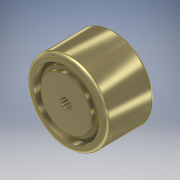
# Autodesk Inventor part: Kolo
Saved by Autodesk Inventor 2017 (Build 210142000, 142)
## iProperties
Created: 2016-11-09
Part Number: Kolo
Material: Generic
Document SubType Name: Modeling
Designer: Shichi
Density: 1 g/cm^3
Appearance: Gold - Metal
Author: Shichi
Autodesk Inventor part; units mm, degrees
ref_plane "YZ Plane" through (0, 0, 0) normal (1, 0, 0) x (0, 1, 0)
ref_plane "XZ Plane" through (0, 0, 0) normal (0, 1, 0) x (-1, 0, 0)
ref_plane "XY Plane" through (0, 0, 0) normal (0, 0, 1) x (1, 0, 0)
sketch "Sketch1" plane through (0, 0, 0) normal (0, 1, 0) x (-1, 0, 0)
  circle A0 centre (0, 0) radius 11
  circle A1 centre (0, 0) radius 1.5
  circle A2 centre (0, 0) radius 2
  circle A3 centre (0, 0) radius 8
  circle A4 centre (0, 0) radius 7
  circle A5 centre (0, 0) radius 9
  dimension "d0" = 22
  dimension "d5" = 3
  dimension "d8" = 4
  dimension "d14" = 16
  dimension "d15" = 14
  dimension "d16" = 18
  constraints: 6 centre point, 6 coincident
  measures "d0" diameter of A0
  measures "d5" diameter of A1
  measures "d8" diameter of A2
  measures "d14" diameter of A3
  measures "d15" diameter of A4
  measures "d16" diameter of A5
extrude "Extrusion1" add sketch "Sketch1" along normal blind 13.2 contours A0 | A1 | A2 | A3 | A4 | A5
shell "Shell1" thickness 2 removed faces 1 at (3.2467, 13.2, -1.704)
fillet "Fillet1" radius 0.5 3 edges at (11, 13.2, 0) (9, 13.2, 0) (11, 0, 0)
extrude "Extrusion2" cut sketch "Sketch1" along normal through all contours A1
extrude "Extrusion3" add sketch "Sketch1" along normal blind 5 contours A0 | A3 | A4 | A5
extrude "Extrusion4" add sketch "Sketch1" along normal blind 13.2 contours A2
fillet "Fillet2" radius 1 1 edges at (11, 0, 0)
extrude "Extrusion5" cut sketch "Sketch1" along normal blind 1 contours A3
extrude "Extrusion6" cut sketch "Sketch1" along normal blind 2 contours A5
body "Solid1"
